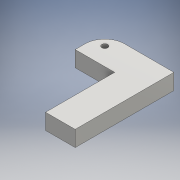
# Autodesk Inventor part: lever_support
Saved by Autodesk Inventor 2016 (Build 200138000, 138)
## iProperties
Created: 2016-04-18
Part Number: lever_support
Material: PC/ABS Plastic
Document SubType Name: Modeling
Designer: amenoni
Density: 0.357273 g/cm^3
Appearance: Smooth - White
Author: amenoni
Autodesk Inventor part; units mm, degrees
ref_plane "YZ Plane" through (0, 0, 0) normal (1, 0, 0) x (0, 1, 0)
ref_plane "XZ Plane" through (0, 0, 0) normal (0, 1, 0) x (-1, 0, 0)
ref_plane "XY Plane" through (0, 0, 0) normal (0, 0, 1) x (1, 0, 0)
sketch "Sketch2" plane through (0, 0, 0) normal (0, 1, 0) x (-1, 0, 0)
  line L0 (-7.5, -4) -> (7.5, -4)
  line L1 (7.5, -4) -> (7.5, 4)
  line L2 (7.5, 4) -> (-7.5, 4)
  line L3 (-7.5, 4) -> (-7.5, -4)
  line L4 (-7.5, -4) -> (7.5, 4) construction
  line L5 (7.5, -4) -> (-7.5, 4) construction
  point P0 (0, 0)
  dimension "d5" = 15
  dimension "d6" = 8
  constraints: 12 end point, 2 midpoint, 2 parallel, 1 horizontal, 1 perpendicular
  measures "d5" distance of L2.end L1.end
  measures "d6" distance of L1.end L0.end
extrude "Extrusion2" add sketch "Sketch2" along normal blind 50
sketch "Sketch3" plane through (-7.5, 0, -4) normal (-1, 0, 0) x (0, 0, 1)
  line L0 (8, 0) -> (8, 50) projected
  line L1 (0, 50) -> (8, 50)
  line L2 (8, 50) -> (8, 35)
  line L3 (8, 35) -> (0, 35)
  line L4 (0, 35) -> (0, 50)
  point P0 (4, 0)
  dimension "d9" = 15
  constraints: 8 end point, 2 parallel, 1 horizontal, 1 perpendicular, 1 point on line
  measures "d9" distance of L1.end L2.end
extrude "Extrusion3" add sketch "Sketch3" along normal blind 20
fillet "Fillet1" radius 10 1 edges at (-27.5, 50, 0)
sketch "Sketch5" plane through (-7.5, 0, 4) normal (0, 0, 1) x (1, 0, 0)
  line L0 (-20, 35) -> (-20, 40) projected
  line L1 (15, 50) -> (-10, 50) projected
  point P0 (7.5, 0)
  point P1 (-14, 44)
  dimension "d13" = 6
  dimension "d14" = 6
  measures "d13" distance from line of L0 point (-14, 44)
  measures "d14" distance from line of point (-14, 44) L1
hole "Hole1" at (-21.5, 44, 4) direction (0, 0, -1) diameter 3 end through all
body "Solid2"
